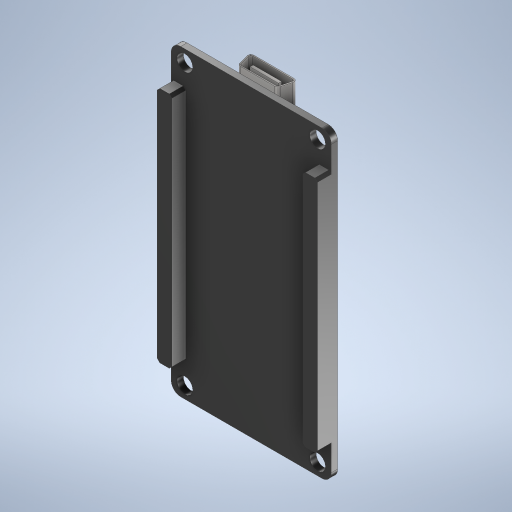
# Autodesk Inventor part: esp32s
Saved by Autodesk Inventor 2023 (Build 270158000, 158)
## iProperties
Created: 2022-06-15
Part Number: esp32s
Material: 일반
Document SubType Name: Modeling
Designer: user
Density: 1 g/cm^3
Appearance: 기본값
Author: user
Autodesk Inventor part; units mm, degrees
ref_plane "YZ Plane" through (0, 0, 0) normal (1, 0, 0) x (0, 1, 0)
ref_plane "XZ Plane" through (0, 0, 0) normal (0, 1, 0) x (-1, 0, 0)
ref_plane "XY Plane" through (0, 0, 0) normal (0, 0, 1) x (1, 0, 0)
sketch "스케치1" plane through (0, 0, 0) normal (0, 0, 1) x (1, 0, 0)
  line L0 (-11.165, 24) -> (11.165, 24)
  line L1 (12.665, 22.5) -> (12.665, -22.5)
  line L2 (11.165, -24) -> (-11.165, -24)
  line L3 (-12.665, -22.5) -> (-12.665, 22.5)
  line L4 (-12.665, 24) -> (12.665, -24) construction
  line L5 (12.665, 24) -> (-12.665, -24) construction
  circle A0 centre (-10.5, 22.1) radius 1.25
  line L6 (0, 0) -> (0, 13.0962) construction
  line L7 (0, 0) -> (6.3269, 0)
  circle A1 centre (10.5, 22.1) radius 1.25
  circle A2 centre (-10.5, -22.1) radius 1.25
  circle A3 centre (10.5, -22.1) radius 1.25
  arc A4 (-11.165, 24) -> (-12.665, 22.5) centre (-11.165, 22.5) ccw
  arc A5 (12.665, 22.5) -> (11.165, 24) centre (11.165, 22.5) ccw
  arc A6 (11.165, -24) -> (12.665, -22.5) centre (11.165, -22.5) ccw
  arc A7 (-12.665, -22.5) -> (-11.165, -24) centre (-11.165, -22.5) ccw
  dimension "d0" = 25.33
  dimension "d1" = 48
  dimension "d2" = 2.5
  dimension "d3" = 1.9
  dimension "d6" = 21
  dimension "d9" = 1.5
  constraints: 16 end point, 8 centre point, 8 point on circle, 8 point on line, 8 tangent, 3 equal radius, 3 symmetric about line, 2 midpoint, 2 parallel, 2 perpendicular, 1 horizontal, 1 vertical, 3 other
  measures "d0" distance of L4.end L5.end
  measures "d1" distance of L5.start L4.end
  measures "d2" diameter of A0
  measures "d3" distance from line of L0 A0.centre
  measures "d6" distance of A1.centre A0.centre
  measures "d9" radius of A4
extrude "돌출1" add sketch "스케치1" along normal blind 1
sketch "스케치2" plane through (-11.165, 24, 0) normal (0, 1, 0) x (1, 0, 0)
  line L0 (8.0166, 2.6) -> (14.3134, 2.6)
  line L1 (14.965, 2.6) -> (14.965, 0)
  line L2 (13.8847, 0) -> (8.4453, 0)
  line L3 (7.365, 0) -> (7.365, 2.6)
  line L4 (7.365, 2.6) -> (14.965, 0) construction
  line L5 (14.965, 2.6) -> (7.365, 0) construction
  line L6 (22.33, 0) -> (0, 0) projected
  line L7 (7.5336, 1.9706) -> (7.9624, 0.3706)
  line L8 (11.165, 1.3) -> (11.165, 2.6) construction
  line L9 (14.7964, 1.9706) -> (14.3676, 0.3706)
  arc A0 (8.0166, 2.6) -> (7.5336, 1.9706) centre (8.0166, 2.1) ccw
  arc A1 (14.7964, 1.9706) -> (14.3134, 2.6) centre (14.3134, 2.1) ccw
  arc A2 (13.8847, 0) -> (14.3676, 0.3706) centre (13.8847, 0.5) ccw
  arc A3 (7.9624, 0.3706) -> (8.4453, 0) centre (8.4453, 0.5) ccw
  line L10 (14.3134, 2.4) -> (8.0166, 2.4)
  arc A4 (8.0166, 2.4) -> (7.7268, 2.0224) centre (8.0166, 2.1) ccw
  line L11 (7.7268, 2.0224) -> (8.1556, 0.4224)
  arc A5 (8.1556, 0.4224) -> (8.4453, 0.2) centre (8.4453, 0.5) ccw
  line L12 (8.4453, 0.2) -> (13.8847, 0.2)
  arc A6 (13.8847, 0.2) -> (14.1744, 0.4224) centre (13.8847, 0.5) ccw
  line L13 (14.1744, 0.4224) -> (14.6032, 2.0224)
  arc A7 (14.6032, 2.0224) -> (14.3134, 2.4) centre (14.3134, 2.1) ccw
  point P0 (11.165, 0)
  point P1 (11.165, 0)
  point P2 (8.0617, 0)
  point P3 (14.2683, 0)
  dimension "d0" = 25.33
  dimension "d1" = 48
  dimension "d2" = 2.5
  dimension "d3" = 1.9
  dimension "d6" = 21
  dimension "d9" = 1.5
  dimension "d10" = 7.6
  dimension "d11" = 2.6
  dimension "d12" = 15
  dimension "d13" = 0.5
  dimension "d14" = 0.5
  dimension "d15" = 0.2
  constraints: 26 end point, 16 point on circle, 9 point on line, 8 centre point, 8 tangent, 5 midpoint, 3 parallel, 2 equal radius, 1 horizontal, 1 perpendicular, 1 symmetric about line, 7 other
  measures "d10" distance of L1.end L3.start
  measures "d11" distance of L1.start L1.end
  measures "d12" angle of L3 L7
  measures "d13" radius of A0
  measures "d14" radius of A1
  measures "d15" distance between parallel lines of L0 L10
extrude "돌출2" add sketch "스케치2" along normal blind 1 and the other way blind 5.6
sketch "스케치3" plane through (-11.165, 18.4, 0) normal (0, -1, 0) x (1, 0, 0)
  arc A0 (8.4453, 0) -> (7.9624, -0.3706) centre (8.4453, -0.5) ccw projected
  line L0 (7.9624, -0.3706) -> (7.5336, -1.9706) projected
  arc A1 (7.5336, -1.9706) -> (8.0166, -2.6) centre (8.0166, -2.1) ccw projected
  line L1 (8.0166, -2.6) -> (14.3134, -2.6) projected
  arc A2 (14.3134, -2.6) -> (14.7964, -1.9706) centre (14.3134, -2.1) ccw projected
  line L2 (14.7964, -1.9706) -> (14.3676, -0.3706) projected
  arc A3 (14.3676, -0.3706) -> (13.8847, 0) centre (13.8847, -0.5) ccw projected
  line L3 (8.4453, 0) -> (13.8847, 0) projected
  arc A4 (14.3134, -2.4) -> (14.6032, -2.0224) centre (14.3134, -2.1) ccw projected
  line L4 (14.3134, -2.4) -> (8.0166, -2.4) projected
  arc A5 (7.7268, -2.0224) -> (8.0166, -2.4) centre (8.0166, -2.1) ccw projected
  line L5 (7.7268, -2.0224) -> (8.1556, -0.4224) projected
  arc A6 (8.4453, -0.2) -> (8.1556, -0.4224) centre (8.4453, -0.5) ccw projected
  line L6 (8.4453, -0.2) -> (13.8847, -0.2) projected
  arc A7 (14.1744, -0.4224) -> (13.8847, -0.2) centre (13.8847, -0.5) ccw projected
  line L7 (14.1744, -0.4224) -> (14.6032, -2.0224) projected
  point P0 (11.165, 0)
  dimension "d0" = 25.33
  dimension "d1" = 48
  dimension "d2" = 2.5
  dimension "d3" = 1.9
  dimension "d6" = 21
  dimension "d9" = 1.5
extrude "돌출3" add sketch "스케치3" against normal blind 1 contours L4 A5 L5 A6 L6 A7 L7 A4
sketch "스케치4" plane through (-11.165, 19.4, 0) normal (0, 1, 0) x (1, 0, 0)
  line L0 (8.0166, 2.4) -> (14.3134, 2.4) projected
  arc A0 (8.0166, 2.4) -> (7.7268, 2.0224) centre (8.0166, 2.1) ccw projected
  line L1 (8.1556, 0.4224) -> (7.7268, 2.0224) projected
  arc A1 (8.1556, 0.4224) -> (8.4453, 0.2) centre (8.4453, 0.5) ccw projected
  line L2 (13.8847, 0.2) -> (8.4453, 0.2) projected
  arc A2 (13.8847, 0.2) -> (14.1744, 0.4224) centre (13.8847, 0.5) ccw projected
  line L3 (14.6032, 2.0224) -> (14.1744, 0.4224) projected
  arc A3 (14.6032, 2.0224) -> (14.3134, 2.4) centre (14.3134, 2.1) ccw projected
  line L4 (8.0166, 2.4) -> (14.3134, 2.4) projected
  line L5 (11.165, 2.4) -> (11.165, 0.2)
  line L6 (13.8847, 0.2) -> (8.4453, 0.2) projected
  line L7 (8.915, 1.05) -> (13.415, 1.05)
  line L8 (13.415, 1.05) -> (13.415, 1.55)
  line L9 (13.415, 1.55) -> (8.915, 1.55)
  line L10 (8.915, 1.55) -> (8.915, 1.05)
  line L11 (8.915, 1.05) -> (13.415, 1.55) construction
  line L12 (13.415, 1.05) -> (8.915, 1.55) construction
  point P0 (11.165, 0)
  point P1 (11.165, 1.3)
  dimension "d0" = 25.33
  dimension "d1" = 48
  dimension "d2" = 2.5
  dimension "d3" = 1.9
  dimension "d6" = 21
  dimension "d9" = 1.5
  dimension "d22" = 4.5
  dimension "d23" = 0.5
  constraints: 14 end point, 5 midpoint, 2 parallel, 1 horizontal, 1 perpendicular
  measures "d22" distance of L9.end L8.end
  measures "d23" distance of L8.end L7.end
extrude "돌출4" add sketch "스케치4" along normal blind 5.25 contours L9 L8 L7 L5 | L5 L7 L10 L9
sketch "스케치5" plane through (0, 0, 0) normal (0, 0, -1) x (-1, 0, 0)
  line L0 (8, 0) -> (-8, 0)
  line L1 (-8, 0) -> (-8, -24)
  line L2 (-8, -24) -> (8, -24)
  line L3 (8, -24) -> (8, 0)
  line L4 (8, 0) -> (-8, -24) construction
  line L5 (-8, 0) -> (8, -24) construction
  line L6 (11.165, -24) -> (-11.165, -24) projected
  line L7 (8, -16) -> (-8, -16)
  line L8 (-8, -16) -> (-8, 0)
  line L9 (-8, 0) -> (8, 0)
  line L10 (8, 0) -> (8, -16)
  line L11 (8, -16) -> (-8, 0) construction
  line L12 (-8, -16) -> (8, 0) construction
  line L13 (-7.8, -15.8) -> (7.8, -15.8)
  line L14 (7.8, -15.8) -> (7.8, -0.2)
  line L15 (7.8, -0.2) -> (-7.8, -0.2)
  line L16 (-7.8, -0.2) -> (-7.8, -15.8)
  point P0 (0, 0)
  point P1 (0, -12)
  point P2 (0, -8)
  point P3 (0, 0)
  dimension "d26" = 24
  dimension "d27" = 16
  dimension "d28" = 16
  dimension "d49" = 0.2
  constraints: 32 end point, 6 midpoint, 6 parallel, 3 perpendicular, 2 horizontal, 2 point on line, 1 vertical alignment, 3 other
  measures "d26" distance of L0.end L1.end
  measures "d27" distance of L1.end L2.end
  measures "d28" distance between parallel lines of L9 L7
  measures "d49" distance between parallel lines of L7 L13
extrude "돌출5" add sketch "스케치5" along normal blind 0.66 contours L3 L7 L1 L0 | L3 L2 L1 L7 | L16 L15 L14 L13
extrude "돌출6" add sketch "스케치5" along normal blind 2.7 contours L16 L15 L14 L13
fillet "모깎기1" radius 0.2 2 edges at (8, -24, -0.33) (-8, -24, -0.33)
sketch "스케치6" plane through (0, 0, -0.66) normal (0, 0, -1) x (-1, 0, 0)
  line L0 (7.2056, -18.287) -> (7.2056, -23.3297)
  line L1 (7.2056, -23.3297) -> (2.3744, -23.3297)
  line L2 (2.3744, -23.3297) -> (2.3744, -19.6975)
  line L3 (2.3744, -19.6975) -> (0.1881, -19.6975)
  line L4 (0.1881, -19.6975) -> (0.1881, -23.3297)
  line L5 (0.1881, -23.3297) -> (-3.1268, -23.3297)
  line L6 (-3.1268, -23.3297) -> (-3.1268, -19.6975)
  line L7 (-3.1268, -19.6975) -> (-5.0663, -19.6975)
  line L8 (-5.0663, -19.6975) -> (-5.0663, -23.3297)
  line L9 (-5.0663, -23.3297) -> (-7.3232, -23.3297)
  line L10 (-7.3232, -23.3297) -> (-7.3232, -18.287)
  line L11 (8, -16) -> (-8, -16)
  line L12 (-6.8232, -18.287) -> (-6.8232, -22.8297)
  line L13 (-6.8232, -22.8297) -> (-5.5663, -22.8297)
  line L14 (-5.5663, -22.8297) -> (-5.5663, -19.1975)
  line L15 (-5.5663, -19.1975) -> (-2.6268, -19.1975)
  line L16 (-2.6268, -19.1975) -> (-2.6268, -22.8297)
  line L17 (-2.6268, -22.8297) -> (-0.3119, -22.8297)
  line L18 (-0.3119, -22.8297) -> (-0.3119, -19.1975)
  line L19 (-0.3119, -19.1975) -> (2.8744, -19.1975)
  line L20 (2.8744, -19.1975) -> (2.8744, -22.8297)
  line L21 (2.8744, -22.8297) -> (6.7056, -22.8297)
  line L22 (6.7056, -22.8297) -> (6.7056, -18.287)
  line L23 (7.2056, -18.287) -> (6.7056, -18.287)
  line L24 (-6.8232, -18.287) -> (-7.3232, -18.287)
  point P0 (0, 0)
  point P1 (7.8, -16)
  point P2 (-7.8, -16)
  dimension "d34" = 0.5
  constraints: 50 end point, 13 perpendicular, 6 point on line, 2 horizontal, 1 vertical, 10 other
  measures "d34" distance between parallel lines of L1 L21
extrude "돌출7" cut sketch "스케치6" against normal blind 0.1
sketch "스케치7" plane through (0, 0, 1) normal (0, 0, 1) x (1, 0, 0)
  line L0 (-12.265, 18.8) -> (-10.765, 18.8)
  line L1 (-10.365, 18.4) -> (-10.365, -18.4)
  line L2 (-10.765, -18.8) -> (-12.265, -18.8)
  line L3 (-12.665, -18.4) -> (-12.665, 18.4)
  line L4 (-12.665, 18.8) -> (-10.365, -18.8) construction
  line L5 (-10.365, 18.8) -> (-12.665, -18.8) construction
  line L6 (-12.665, 22.5) -> (-12.665, -22.5) projected
  line L7 (-10.765, 18.8) -> (-10.365, 18.4)
  line L8 (-12.265, 18.8) -> (-12.665, 18.4)
  line L9 (-10.365, -18.4) -> (-10.765, -18.8)
  line L10 (-12.265, -18.8) -> (-12.665, -18.4)
  point P0 (0, 0)
  point P1 (-11.515, 0)
  point P2 (-12.665, 0)
  dimension "d37" = 37.6
  dimension "d38" = 2.3
  dimension "d41" = 0.4
  dimension "d42" = 0.4
  dimension "d43" = 0.4
  dimension "d44" = 0.4
  dimension "d45" = 0.4
  dimension "d46" = 0.4
  dimension "d47" = 0.4
  dimension "d48" = 0.4
  constraints: 20 end point, 8 point on line, 4 midpoint, 2 parallel, 1 horizontal, 1 perpendicular
  measures "d37" distance of L5.start L4.end
  measures "d38" distance of L4.start L5.start
  measures "d41" distance of L0.end L5.start
  measures "d42" distance of L1.start L5.start
  measures "d43" distance of L0.start L4.start
  measures "d44" distance of L3.end L4.start
  measures "d45" distance of L1.end L4.end
  measures "d46" distance of L2.start L4.end
  measures "d47" distance of L2.end L5.end
  measures "d48" distance of L3.start L5.end
extrude "돌출8" add sketch "스케치7" along normal blind 2.2
mirror "미러1" about plane through (0, 0, 0) normal (1, 0, 0) of "돌출8"
fillet "모깎기2" radius 0.2 4 edges at (-7.8, -0.2, -1.68) (7.8, -0.2, -1.68) (-7.8, -15.8, -1.68) (7.8, -15.8, -1.68)
equation "\"d42\" = d41"
equation "\"d43\" = d41"
equation "\"d44\" = d43"
equation "\"d45\" = d41"
equation "\"d46\" = d45"
equation "\"d47\" = d41"
equation "\"d48\" = d47"
